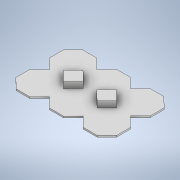
# Autodesk Inventor part: TokenHolderLid
Saved by Autodesk Inventor 2020 (Build 240168000, 168)
## iProperties
Created: 2020-06-18
Part Number: TokenHolderLid
Material: Generic
Document SubType Name: Modeling
Designer: user
Density: 1 g/cm^3
Appearance: Default
Author: user
## iProperties of the stored document _3DPrint.ipt
Created: 2020-06-18
Part Number: _3DPrint
Material: Generic
Document SubType Name: Modeling
Designer: user
Density: 1 g/cm^3
Appearance: Default
Author: user
Autodesk Inventor part; units mm, degrees
ref_plane "YZ Plane" through (0, 0, 0) normal (1, 0, 0) x (0, 1, 0)
ref_plane "XZ Plane" through (0, 0, 0) normal (0, 1, 0) x (-1, 0, 0)
ref_plane "XY Plane" through (0, 0, 0) normal (0, 0, 1) x (1, 0, 0)
sketch "Sketch1" plane through (0, 0, 0) normal (0, 1, 0) x (-1, 0, 0)
  line L0 (-9.0015, 10.4204) -> (-9.0261, 19.4984)
  line L1 (-9.0261, 19.4984) -> (-2.6244, 25.9349)
  line L2 (-2.6244, 25.9349) -> (6.4536, 25.9595)
  line L3 (6.4536, 25.9595) -> (12.8901, 19.5578)
  line L4 (12.8901, 19.5578) -> (12.9147, 10.4798)
  line L5 (12.9147, 10.4798) -> (6.513, 4.0433)
  line L6 (6.513, 4.0433) -> (-2.565, 4.0187)
  line L7 (-2.565, 4.0187) -> (-9.0015, 10.4204)
  line L8 (-2.565, 4.0187) -> (-8.9493, -2.4351)
  line L9 (-8.9493, -2.4351) -> (-15.4031, 3.9491)
  line L10 (-15.4031, 3.9491) -> (-9.0015, 10.4204)
  line L11 (-8.9667, -2.4178) -> (-8.9421, -11.4958)
  line L12 (-8.9421, -11.4958) -> (-2.5056, -17.8975)
  line L13 (-2.5056, -17.8975) -> (6.5724, -17.8729)
  line L14 (6.5724, -17.8729) -> (12.9741, -11.4364)
  line L15 (12.9741, -11.4364) -> (12.9495, -2.3584)
  line L16 (12.9495, -2.3584) -> (6.513, 4.0433)
  line L17 (-24.4812, 3.9593) -> (-15.4032, 3.9839)
  line L18 (-30.883, -2.4772) -> (-24.4812, 3.9593)
  line L19 (-30.8584, -11.5552) -> (-30.883, -2.4772)
  line L20 (-24.4219, -17.9569) -> (-30.8584, -11.5552)
  line L21 (-15.3439, -17.9323) -> (-24.4219, -17.9569)
  line L22 (-8.9421, -11.4958) -> (-15.3439, -17.9323)
  line L23 (-30.9178, 10.361) -> (-24.4812, 3.9593)
  line L24 (-30.9423, 19.439) -> (-30.9178, 10.361)
  line L25 (-24.5406, 25.8755) -> (-30.9423, 19.439)
  line L26 (-15.4626, 25.9001) -> (-24.5406, 25.8755)
  line L27 (-9.0261, 19.4984) -> (-15.4626, 25.9001)
  line L28 (-52.834, 10.3017) -> (-52.8586, 19.3797)
  line L29 (-52.8166, -2.554) -> (-46.3975, 3.8652)
  line L30 (-46.3975, 3.8652) -> (-52.834, 10.3017)
  line L31 (-52.7992, -2.5366) -> (-52.7746, -11.6146)
  line L32 (-37.3195, 3.9245) -> (-46.3975, 3.8999)
  line L33 (-30.883, -2.4772) -> (-37.3195, 3.9245)
  line L34 (-37.2601, -17.9917) -> (-30.8584, -11.5552)
  line L35 (-46.3381, -18.0163) -> (-37.2601, -17.9917)
  line L36 (-52.7746, -11.6146) -> (-46.3381, -18.0163)
  line L37 (-30.9178, 10.361) -> (-37.3195, 3.9245)
  line L38 (-37.3789, 25.8408) -> (-30.9423, 19.439)
  line L39 (-46.4569, 25.8162) -> (-37.3789, 25.8408)
  line L40 (-52.8586, 19.3797) -> (-46.4569, 25.8162)
  point P0 (0, 0)
  point P1 (1.9443, 14.9891)
  dimension "d0" = 9.078
  dimension "d3" = 9.078
  dimension "d4" = 9.078
  constraints: 82 end point, 2 perpendicular, 1 symmetric about line, 17 other
  measures "d0" vertical distance of L3.end L4.end
  measures "d3" distance of L6.end L8.end
  measures "d4" distance of L8.end L9.end
extrude "Extrusion1" add sketch "Sketch1" along normal blind 1 contours L10 L9 L11 L22 L21 L20 L19 L18 L23 L24 L25 L26 L27 L0 | L0 L1 L2 L3 L4 L5 L6 L7 | L6 L16 L15 L14 L13 L12 L11 L9 L8 | L24 L37 L33 L19 L34 L35 L36 L31 L29 L30 L28 L40 L39 L38
extrude "Extrusion2" add sketch "Sketch1" along normal blind 5 contours L7 L8 L9 L10 | L23 L18 L33 L37
body "Solid1"
